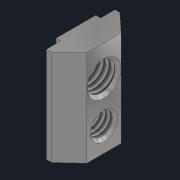
# Autodesk Inventor part: HNTC5_n
Saved by Autodesk Inventor 2022 (Build 260153000, 153)
## iProperties
Part Number: HNTC5_n
Material: 鋼、炭素鋼
Catalog Web Link: www.cadenas.de
Description: HNTC_nut-Nuts for Aluminum Extrusions - Pre-Assembly Fitting Lock Nuts - Nut
Vendor: MISUMI
Document SubType Name: Modeling
Designer: partserver
Manufacturer: MISUMI
Mass: 2.71569 g
Surface Area: 4.56492 cm^2
Volume: 0.345948 cm^3
Density: 7.85 g/cm^3
Appearance: 半つや出し
Category: PARTsolutions
Company: MISUMI
PSOL_IDENT_0: {$CADENAS_DATA\23d-libs\misumi\metric\38_al_extrusions_blackets\nuts\hntc5\hntc.prj},154 {VTYP=3D},{
PSOL_IDENT_1: NB=HNTC5_n},{LINA=HNTC5},{NN=HNTC_nut},{DATE=28.07.2021 09:30:12},{GEOMDATE=13.02.2017 04:04:54},{VE
PSOL_IDENT_2: RSION=},{LINEID=10},{WBVAR=},{WBNUMERIC=}  {NB=HNTC5_n},{LINA=HNTC5},{KT=DUMMY},{PN=HNTC5},{TYPE=HNT
PSOL_IDENT_3: C},{MAT=1010 Carbon Steel or Equivalent},{ST=Trivalent Chromate},{M=5},{RTT=6.8},{B=10.000},{L=14.00
PSOL_IDENT_4: 0},{L1=3.500},{L2=4.500},{A=5.800},{E=3.400},{T=4.100},{W=5.000},{R1=0.000},{R2=0.000},{F=43.000},{L
PSOL_IDENT_5: S=4.000}
NB: HNTC5_n
NN: HNTC_nut
NT: Nuts for Aluminum Extrusions - Pre-Assembly Fitting Lock Nuts - Nut
NBSYN: $PN._n
LINA: HNTC5
CATALOG: Misumi
MAT: 1010 Carbon Steel or Equivalent
ST: Trivalent Chromate
M: 5
RTT: 6.8
B: 10
L: 14
L1: 3.5
L2: 4.5
A: 5.8
E: 3.4
T: 4.1
W: 5
R1: 0
R2: 0
F: 43
LS: 4
SUPPLIER: MISUMI
ARTICLENO: HNTC5_n
BOMINFO: HNTC5
CREATOR: CADENAS GmbH
Title: HNTC5
Author: Cadenas PARTsolutions
Comments: Nuts for Aluminum Extrusions - Pre-Assembly Fitting Lock Nuts - Nut
Autodesk Inventor part; units mm, degrees
sketch "Sketch_1" plane through (0, 0, 0) normal (0, 0, 1) x (1, 0, 0)
  line L0 (-4.1, -2.5) -> (-1.4191, -5)
  line L1 (-1.4191, -5) -> (-0.7, -5)
  line L2 (-0.7, -5) -> (-0.7, -2.9)
  line L3 (-0.7, -2.9) -> (0, -2.9)
  line L4 (0, -2.9) -> (0, 2.9)
  line L5 (0, 2.9) -> (-0.7, 2.9)
  line L6 (-0.7, 2.9) -> (-0.7, 5)
  line L7 (-0.7, 5) -> (-1.4191, 5)
  line L8 (-1.4191, 5) -> (-4.1, 2.5)
  line L9 (-4.1, 2.5) -> (-4.1, -2.5)
  constraints: 20 end point
extrude "Extrusion1" add sketch "Sketch_1" against normal blind 14
sketch "Sketch_2" plane through (0, 0, -3.5) normal (0, 0, 1) x (1, 0, 0)
  line L0 (0, 0) -> (-4.1, 0)
  line L1 (-4.1, 0) -> (-4.1, 2)
  line L2 (-4.1, 2) -> (-3.721, 1.621)
  line L3 (-3.721, 1.621) -> (-0.379, 1.621)
  line L4 (-0.379, 1.621) -> (0, 2)
  line L5 (0, 2) -> (0, 0)
  line L6 (0, 0) -> (-4.1, 0)
  constraints: 14 end point
revolve "Revolution1" cut sketch "Sketch_2" angle 360 about axis through (0, 0, -3.5) along (1, 0, 0)
thread "Thread1" size "M4x0.7" class "6H" standard "ISO Metric profile" full length
sketch "Sketch_3" plane through (0, 0, -9.5) normal (0, 0, 1) x (1, 0, 0)
  line L0 (0, 0) -> (-4.1, 0)
  line L1 (-4.1, 0) -> (-4.1, 2.5)
  line L2 (-4.1, 2.5) -> (-3.667, 2.067)
  line L3 (-3.667, 2.067) -> (-0.433, 2.067)
  line L4 (-0.433, 2.067) -> (0, 2.5)
  line L5 (0, 2.5) -> (0, 0)
  line L6 (0, 0) -> (-4.1, 0)
  constraints: 14 end point
revolve "Revolution2" cut sketch "Sketch_3" angle 360 about axis through (0, 0, -9.5) along (1, 0, 0)
thread "Thread2" size "M5x0.8" class "6H" standard "ISO Metric profile" full length
ref_plane "bolt_XY" through (-4.1, 0, -9.5) normal (1, 0, 0) x (0, 0, -1)
ref_plane "bolt_YZ" through (-4.1, 0, -9.5) normal (0, 0, -1) x (0, 1, 0)
ref_plane "bolt_ZX" through (-4.1, 0, -9.5) normal (0, 1, 0) x (1, 0, 0)
ref_plane "frame_XY" through (-0.7, 0, -9.5) normal (1, 0, 0) x (0, 0, -1)
ref_plane "frame_YZ" through (-0.7, 0, -9.5) normal (0, 0, -1) x (0, 1, 0)
ref_plane "frame_ZX" through (-0.7, 0, -9.5) normal (0, 1, 0) x (1, 0, 0)
ref_plane "nut_XY" through (0, 0, -9.5) normal (1, 0, 0) x (0, 0, -1)
ref_plane "nut_YZ" through (0, 0, -9.5) normal (0, 0, -1) x (0, 1, 0)
ref_plane "nut_ZX" through (0, 0, -9.5) normal (0, 1, 0) x (1, 0, 0)
ref_plane "set_screw_XY" through (-4.1, 0, -3.5) normal (1, 0, 0) x (0, 0, -1)
ref_plane "set_screw_YZ" through (-4.1, 0, -3.5) normal (0, 0, -1) x (0, 1, 0)
ref_plane "set_screw_ZX" through (-4.1, 0, -3.5) normal (0, 1, 0) x (1, 0, 0)
body "Solid1"
